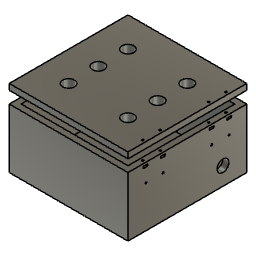
Caja de PF Gaby (Autodesk Fusion 360 design; units mm, degrees)
Autodesk Fusion 360 part; units mm, degrees
note: some values were not read from the file. Set by a fixed rule: which face or edge a step refers to.
sketch "Boceto1" plane through (0, 0, 0) normal (0, 0, 1) x (1, 0, 0)
  line L0 (0, 0) -> (-200, 0)
  line L1 (-200, 0) -> (-200, 200)
  line L2 (-200, 200) -> (0, 200)
  line L3 (0, 200) -> (0, 0)
  dimension "d1" = 200
  dimension "d2" = 200
  constraint horizontal L0
  constraint vertical L1
  constraint horizontal L2
  constraint vertical L3
  constraint coincident L0.start L3.end
  measures "d1" distance of L0.end L1.end
  measures "d2" distance of L0.start L0.end
extrude "Extruir1" add sketch "Boceto1" along normal blind 100 makes body 1
shell "Vaciado1" thickness 10 removed faces 1 at (-66.6667, 66.6667, 100) on bodies 1
sketch "Boceto2" plane through (0, 0, 100) normal (0, 0, 1) x (-1, 0, 0)
  line L0 (10, -190) -> (10, -10)
  line L1 (10, -10) -> (190, -10)
  line L2 (190, -10) -> (190, -190)
  line L3 (190, -190) -> (10, -190)
  line L4 (0, -200) -> (200, -200)
  line L5 (200, -200) -> (200, 0)
  line L6 (200, 0) -> (0, 0)
  line L7 (0, 0) -> (0, -200)
  line L8 (0, 0) -> (200, 0)
  line L9 (200, 0) -> (200, -200)
  line L10 (200, -200) -> (0, -200)
  line L11 (0, -200) -> (0, 0)
  constraint horizontal L8
  constraint vertical L9
  constraint horizontal L10
  constraint vertical L11
  constraint coincident L4.end L5.start
  constraint coincident L6.end L7.start
sketch "Boceto3" plane through (0, 0, 100) normal (0, 0, 1) x (-1, 0, 0)
  line L0 (10, -190) -> (10, -10)
  line L1 (10, -10) -> (190, -10)
  line L2 (190, -10) -> (190, -190)
  line L3 (190, -190) -> (10, -190)
  line L4 (0, -200) -> (200, -200)
  line L5 (200, -200) -> (200, 0)
  line L6 (200, 0) -> (0, 0)
  line L7 (0, 0) -> (0, -200)
  line L8 (200, -200) -> (0, -200)
  line L9 (0, -200) -> (0, 0)
  line L10 (0, 0) -> (200, 0)
  line L11 (200, 0) -> (200, -200)
  constraint horizontal L8
  constraint vertical L9
  constraint horizontal L10
  constraint vertical L11
  constraint coincident L6.end L7.start
  constraint coincident L4.end L5.start
extrude "Extruir3" add sketch "Boceto3" along normal blind 5 separate body contours L0 L1 L2 L3 makes body 2
sketch "Boceto4" plane through (0, 0, 105) normal (0, 0, 1) x (-1, 0, 0)
  line L0 (190, -190) -> (190, -10)
  line L1 (190, -10) -> (10, -10)
  line L2 (10, -10) -> (10, -190)
  line L3 (10, -190) -> (190, -190)
  line L4 (200, -200) -> (0, -200)
  line L5 (0, -200) -> (0, 0)
  line L6 (0, 0) -> (200, 0)
  line L7 (200, 0) -> (200, -200)
  constraint horizontal L4
  constraint vertical L5
  constraint horizontal L6
  constraint vertical L7
  constraint coincident L5.end L6.start
extrude "Extruir4" add sketch "Boceto4" along normal blind 10 separate body contours L0 L1 L2 L3 | L4 L5 L6 L7 makes body 3
combine "Combinar1" operation add target body 3 tool bodies 2
move_body "Desplazar1" bodies 3 to x (1, 0, 0) y (0, 1, 0) z (0, 0, 1) at (0, 0, -5)
sketch "Boceto5" plane through (0, 0, 0) normal (1, 0, 0) x (0, 1, 0)
  line L0 (0, 0) -> (200, 0)
  line L1 (200, 0) -> (200, 100)
  line L2 (200, 100) -> (0, 100)
  line L3 (0, 100) -> (0, 0)
  circle A0 centre (160, 30) radius 10
  dimension "d13" = 20
  dimension "d14" = 30
  dimension "d15" = 40
  measures "d13" diameter of A0
  measures "d14" distance of L0 A0.centre
  measures "d15" distance of L1 A0.centre
extrude "Extruir5" cut sketch "Boceto5" against normal blind 50 contours A0 bodies 1
sketch "Boceto6" plane through (0, 0, 110) normal (0, 0, 1) x (-1, 0, 0)
  line L0 (200, 0) -> (0, 0)
  line L1 (0, 0) -> (0, -200)
  line L2 (0, -200) -> (200, -200)
  line L3 (200, -200) -> (200, 0)
  line L4 (100, -200) -> (100, 0)
  circle A0 centre (150, -100) radius 10
  circle A1 centre (150, -50) radius 10
  circle A2 centre (150, -150) radius 10
  circle A3 centre (50, -50) radius 10
  circle A4 centre (50, -100) radius 10
  circle A5 centre (50, -150) radius 10
  dimension "d18" = 100
  dimension "d19" = 20
  dimension "d20" = 50
  dimension "d21" = 100
  dimension "d22" = 20
  dimension "d23" = 50
  dimension "d26" = 20
  dimension "d27" = 50
  dimension "d29" = 50
  dimension "d30" = 50
  dimension "d31" = 50
  dimension "d32" = 50
  constraint coincident L2 L4.start
  constraint coincident L0 L4.end
  constraint perpendicular L0 L4
  constraint symmetric L4 A0 A4
  constraint symmetric L4 A1 A3
  constraint symmetric L4 A2 A5
  measures "d18" distance of L0.end L4.end
  measures "d19" diameter of A0
  measures "d20" distance of L3 A0.centre
  measures "d21" distance of L0 A0.centre
  measures "d22" diameter of A1
  measures "d23" distance of L3 A1.centre
  measures "d26" diameter of A2
  measures "d27" distance of L3 A2.centre
  measures "d29" distance of L0 A1.centre
  measures "d30" distance of L2 A2.centre
  measures "d31" distance of A0.centre A1.centre
  measures "d32" distance of A0.centre A2.centre
extrude "Extruir6" cut sketch "Boceto6" against normal blind 75 contours A0 | A1 | A2 | A3 | A4 | A5 bodies 3
sketch "Boceto7" plane through (0, 0, 110) normal (0, 0, 1) x (-1, 0, 0)
  circle A0 centre (150, -150) radius 10
  circle A1 centre (50, -50) radius 10
  circle A2 centre (150, -100) radius 10
  circle A3 centre (50, -150) radius 10
  circle A4 centre (50, -100) radius 10
  circle A5 centre (150, -50) radius 10
  line L0 (200, 0) -> (0, 0)
  line L1 (0, 0) -> (0, -200)
  line L2 (0, -200) -> (200, -200)
  line L3 (200, -200) -> (200, 0)
  circle A6 centre (5, -30) radius 1.6
  line L4 (10, -190) -> (10, -10)
  circle A7 centre (5, -59) radius 1.6
  line L5 (200, -100) -> (0, -100)
  circle A8 centre (5, -141) radius 1.6
  circle A9 centre (5, -170) radius 1.6
  dimension "d35" = 3.2
  dimension "d36" = 5
  dimension "d37" = 10
  dimension "d38" = 30
  dimension "d39" = 3.2
  dimension "d40" = 29
  dimension "d41" = 200
  dimension "d42" = 200
  dimension "d57" = 59
  constraint coincident L3 L5.start
  constraint coincident L1 L5.end
  constraint perpendicular L1 L5
  constraint symmetric A6 L5 A9
  constraint symmetric A7 L5 A8
  measures "d35" diameter of A6
  measures "d36" distance of L1 A6.centre
  measures "d37" distance of L1 L4
  measures "d38" distance of L0 A6.centre
  measures "d39" diameter of A7
  measures "d40" distance of A6.centre A7.centre
  measures "d41" distance of L0.start L2.end
  measures "d42" distance of L1.end L2.end
  measures "d57" distance of L0 A7.centre
extrude "Extruir7" cut sketch "Boceto7" against normal blind 15 contours A6 | A7 | A8 | A9 bodies 1 3
sketch "Boceto8" plane through (0, 0, 0) normal (1, 0, 0) x (0, 1, 0)
  circle A0 centre (160, 30) radius 10
  line L0 (0, 0) -> (200, 0)
  line L1 (200, 0) -> (200, 100)
  line L2 (200, 100) -> (0, 100)
  line L3 (0, 100) -> (0, 0)
  line L4 (25.5, 96) -> (33.5, 96)
  line L5 (33.5, 96) -> (33.5, 93)
  line L6 (33.5, 93) -> (25.5, 93)
  line L7 (25.5, 93) -> (25.5, 96)
  line L8 (55, 96) -> (63, 96)
  line L9 (63, 96) -> (63, 93)
  line L10 (63, 93) -> (55, 93)
  line L11 (55, 93) -> (55, 96)
  circle A1 centre (30, 70) radius 1.6
  circle A2 centre (59, 70) radius 1.6
  line L12 (100, 100) -> (100, 0)
  line L13 (166.5, 93) -> (174.5, 93)
  line L14 (166.5, 96) -> (166.5, 93)
  line L15 (174.5, 96) -> (166.5, 96)
  line L16 (174.5, 93) -> (174.5, 96)
  line L17 (145, 93) -> (145, 96)
  line L18 (137, 93) -> (145, 93)
  line L19 (137, 96) -> (137, 93)
  line L20 (145, 96) -> (137, 96)
  circle A3 centre (141, 70) radius 1.6
  circle A4 centre (170, 70) radius 1.6
  dimension "d47" = 3
  dimension "d48" = 8
  dimension "d49" = 4
  dimension "d50" = 25.5
  dimension "d52" = 3
  dimension "d53" = 4
  dimension "d54" = 8
  dimension "d56" = 55
  dimension "d61" = 3.2
  dimension "d62" = 30
  dimension "d63" = 30
  dimension "d64" = 3.2
  dimension "d65" = 59
  dimension "d66" = 30
  dimension "d67" = 100
  constraint horizontal L4
  constraint vertical L5
  constraint horizontal L6
  constraint vertical L7
  constraint horizontal L8
  constraint vertical L9
  constraint horizontal L10
  constraint vertical L11
  constraint coincident L2 L12.start
  constraint coincident L0 L12.end
  constraint perpendicular L0 L12
  constraint symmetric L4.start L12 L15.start
  constraint symmetric L4.end L12 L14.start
  constraint symmetric L5.end L12 L13.start
  constraint symmetric L6.end L12 L13.end
  constraint symmetric L8.start L12 L17.end
  constraint symmetric L8.end L12 L19.start
  constraint symmetric L9.end L12 L18.start
  constraint symmetric L10.end L12 L17.start
  constraint symmetric A1 L12 A4
  constraint symmetric A2 L12 A3
  measures "d47" distance of L4.start L6.end
  measures "d48" distance of L5.end L6.end
  measures "d49" distance of L2 L4
  measures "d50" distance of L3 L7
  measures "d52" distance of L8.start L10.end
  measures "d53" distance of L2 L8
  measures "d54" distance of L9.end L10.end
  measures "d56" distance of L3 L11
  measures "d61" diameter of A1
  measures "d62" distance of L3 A1.centre
  measures "d63" distance of L2 A1.centre
  measures "d64" diameter of A2
  measures "d65" distance of L3 A2.centre
  measures "d66" distance of L2 A2.centre
  measures "d67" distance of L3 L12
extrude "Extruir9" cut sketch "Boceto8" against normal up to surface (10 mm away) contours L4 L5 L6 L7 | L8 L9 L10 L11 | A1 | A2 | L13 L14 L15 L16 | L17 L18 L19 L20 | A3 | A4 bodies 1
move_body "Desplazar2" bodies 3 to x (1, 0, 0) y (0, 1, 0) z (0, 0, 1) at (0, 0, 20)
